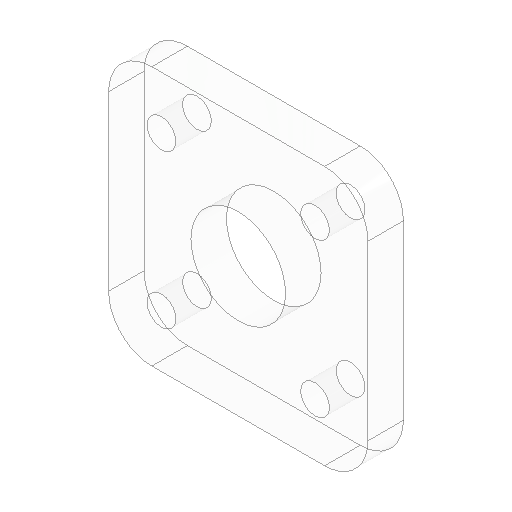
# Autodesk Inventor part: Tope_rodamiento
Saved by Autodesk Inventor 2025.3 (Build 293356000, 356)
## iProperties
Created: 2025-11-11
Part Number: Tope_rodamiento
Material: PMMA Plastic
Document SubType Name: Modeling
Designer: Gabriel Bojaca
Density: 1.188 g/cm^3
Appearance: Polycarbonate - Clear
Author: Gabriel Bojaca
Autodesk Inventor part; units mm, degrees
ref_plane "YZ Plane" through (0, 0, 0) normal (1, 0, 0) x (0, 1, 0)
ref_plane "XZ Plane" through (0, 0, 0) normal (0, 1, 0) x (-1, 0, 0)
ref_plane "XY Plane" through (0, 0, 0) normal (0, 0, 1) x (1, 0, 0)
sketch "Sketch1" plane through (0, 0, 0) normal (0, 0, 1) x (1, 0, 0)
  line L0 (-9, -13.5) -> (9, -13.5)
  line L1 (13.5, -9) -> (13.5, 9)
  line L2 (9, 13.5) -> (-9, 13.5)
  line L3 (-13.5, 9) -> (-13.5, -9)
  line L4 (-13.5, -13.5) -> (13.5, 13.5) construction
  line L5 (13.5, -13.5) -> (-13.5, 13.5) construction
  line L6 (-8, -8) -> (8, -8) construction
  line L7 (8, -8) -> (8, 8) construction
  line L8 (8, 8) -> (-8, 8) construction
  line L9 (-8, 8) -> (-8, -8) construction
  line L10 (-8, -8) -> (8, 8) construction
  line L11 (8, -8) -> (-8, 8) construction
  circle A0 centre (-8, 8) radius 1.5
  circle A1 centre (8, 8) radius 1.5
  circle A2 centre (-8, -8) radius 1.5
  circle A3 centre (8, -8) radius 1.5
  arc A4 (-9, 13.5) -> (-13.5, 9) centre (-9, 9) ccw
  arc A5 (-13.5, -9) -> (-9, -13.5) centre (-9, -9) ccw
  arc A6 (9, -13.5) -> (13.5, -9) centre (9, -9) ccw
  arc A7 (13.5, 9) -> (9, 13.5) centre (9, 9) ccw
  circle A8 centre (0, 0) radius 4.925
  dimension "d0" = 27
  dimension "d1" = 27
  dimension "d2" = 16
  dimension "d3" = 16
  dimension "d4" = 3
  dimension "d5" = 3
  dimension "d6" = 3
  dimension "d7" = 3
  dimension "d8" = 4.5
  dimension "d9" = 9.85
  constraints: 24 end point, 9 centre point, 8 point on circle, 8 point on line, 8 tangent, 5 coincident, 4 midpoint, 4 parallel, 3 equal radius, 2 horizontal, 2 perpendicular
  measures "d0" distance of L5.end L4.end
  measures "d1" distance of L4.end L5.start
  measures "d2" distance of L8.end L7.end
  measures "d3" distance of L7.end L6.end
  measures "d4" diameter of A0
  measures "d5" diameter of A1
  measures "d6" diameter of A2
  measures "d7" diameter of A3
  measures "d8" radius of A4
  measures "d9" diameter of A8
extrude "Extrusion1" add sketch "Sketch1" along normal blind 3.7
body "Solid1"
